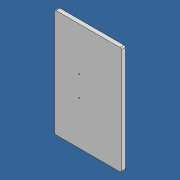
# Autodesk Inventor part: Display
Saved by Autodesk Inventor 2020 (Build 240168000, 168)
## iProperties
Created: 2021-04-28
Part Number: Display
Material: 一般
Document SubType Name: Modeling
Designer: ken113
Density: 1 g/cm^3
Appearance: 既定
Author: ken113
Autodesk Inventor part; units mm, degrees
ref_plane "YZ Plane" through (0, 0, 0) normal (1, 0, 0) x (0, 1, 0)
ref_plane "XZ Plane" through (0, 0, 0) normal (0, 1, 0) x (-1, 0, 0)
ref_plane "XY Plane" through (0, 0, 0) normal (0, 0, 1) x (1, 0, 0)
sketch "スケッチ1" plane through (0, 0, 0) normal (0, 0, 1) x (1, 0, 0)
  line L0 (122.5, -197.5) -> (-122.5, -197.5)
  line L1 (-122.5, -197.5) -> (-122.5, 197.5)
  line L2 (-122.5, 197.5) -> (122.5, 197.5)
  line L3 (122.5, 197.5) -> (122.5, -197.5)
  line L4 (122.5, -197.5) -> (-122.5, 197.5) construction
  line L5 (-122.5, -197.5) -> (122.5, 197.5) construction
  point P0 (0, 0)
  dimension "d0" = 245
  dimension "d1" = 395
  constraints: 12 end point, 2 midpoint, 2 parallel, 1 horizontal, 1 perpendicular
  measures "d0" distance of L1.end L2.end
  measures "d1" distance of L0.end L1.end
extrude "押し出し1" add sketch "スケッチ1" along normal blind 15
sketch "スケッチ2" plane through (0, 0, 15) normal (0, 0, 1) x (1, 0, 0)
  line L0 (-122.5, 197.5) -> (-122.5, -197.5) projected
  line L1 (122.5, 197.5) -> (-122.5, 197.5) projected
  point P0 (0, 0)
  point P1 (-32.5, 37.5)
  point P2 (-32.5, -37.5)
  dimension "d4" = 90
  dimension "d5" = 75
  dimension "d6" = 160
  constraints: 1 vertical alignment
  measures "d4" distance from line of L0 point (-32.5, 37.5)
  measures "d5" distance of point (-32.5, -37.5) point (-32.5, 37.5)
  measures "d6" distance from line of point (-32.5, 37.5) L1
hole "穴1" at (-32.5, 37.5, 15) at (-32.5, -37.5, 15) direction (0, 0, -1) diameter 4.134 depth 6 tip angle 118 thread size "M5x0.8" class "6H" standard "ISO Metric profile"
sketch "スケッチ3" plane through (0, 0, 0) normal (0, 0, -1) x (-1, 0, 0)
  line L0 (122.5, -197.5) -> (-122.5, -197.5) projected
  line L1 (122.5, 197.5) -> (122.5, -197.5) projected
  line L2 (-122.5, 197.5) -> (122.5, 197.5) projected
  line L3 (-122.5, -197.5) -> (-122.5, 197.5) projected
  line L4 (102.5, 192.5) -> (-117.5, 192.5)
  line L5 (-117.5, 192.5) -> (-117.5, -192.5)
  line L6 (-117.5, -192.5) -> (102.5, -192.5)
  line L7 (102.5, -192.5) -> (102.5, 192.5)
  point P0 (0, 0)
  dimension "d14" = 5
  dimension "d15" = 5
  dimension "d16" = 5
  dimension "d17" = 20
  constraints: 8 end point, 2 parallel, 1 horizontal, 1 perpendicular
  measures "d14" distance between parallel lines of L5 L3
  measures "d15" distance between parallel lines of L4 L2
  measures "d16" distance between parallel lines of L0 L6
  measures "d17" distance between parallel lines of L1 L7
extrude "押し出し2" cut sketch "スケッチ3" against normal blind 0.5 contours L7 L6 L5 L4
fillet "フィレット1" radius 5 4 edges at (122.5, -197.5, 7.5) (-122.5, -197.5, 7.5) (122.5, 197.5, 7.5) (-122.5, 197.5, 7.5)
